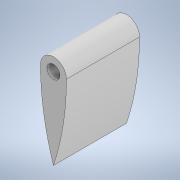
# Autodesk Inventor part: Airfoil
Saved by Autodesk Inventor 2022 (Build 260153000, 153)
## iProperties
Created: 2022-10-13
Part Number: Airfoil
Material: Generic
Document SubType Name: Modeling
Designer: Jasper
Density: 1 g/cm^3
Appearance: Default
Author: Jasper
Autodesk Inventor part; units mm, degrees
ref_plane "YZ Plane" through (0, 0, 0) normal (1, 0, 0) x (0, 1, 0)
ref_plane "XZ Plane" through (0, 0, 0) normal (0, 1, 0) x (-1, 0, 0)
ref_plane "XY Plane" through (0, 0, 0) normal (0, 0, 1) x (1, 0, 0)
sketch "Sketch1" plane through (0, 0, 0) normal (0, 0, 1) x (1, 0, 0)
  arc A0 (8, 0) -> (-8, 0) centre (0, 0) ccw
  arc A1 (0, -50) -> (8, 0) centre (-152.25, 0) ccw
  arc A2 (-8, 0) -> (0, -50) centre (152.25, 0) ccw
  dimension "d0" = 8
  dimension "d2" = 50
  constraints: 6 point on circle, 3 centre point, 2 horizontal alignment, 2 tangent, 1 coincident, 1 vertical alignment
  measures "d0" radius of A0
  measures "d2" distance of A1.start point (0, 0)
extrude "Extrusion1" add sketch "Sketch1" along normal blind 45
sketch "Sketch2" plane through (0, 0, 45) normal (0, 0, 1) x (1, 0, 0)
  point P0 (0, 0)
  point P1 (0, 0)
  constraints: 1 coincident
hole "Hole1" at (0, 0, 45) direction (0, 0, -1) diameter 8 end through all
body "Solid1"
